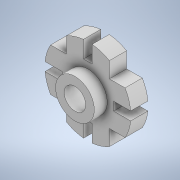
# Autodesk Inventor part: Assignment 3.5 - Indexing Guide
Saved by Autodesk Inventor 2022 (Build 260153000, 153)
## iProperties
Created: 2021-05-24
Part Number: Assignment 3.5 - Indexing Guide
Material: Generic
Document SubType Name: Modeling
Designer: Aaron
Density: 1 g/cm^3
Appearance: Default
Author: Aaron
Autodesk Inventor part; units mm, degrees
ref_plane "YZ Plane" through (0, 0, 0) normal (1, 0, 0) x (0, 1, 0)
ref_plane "XZ Plane" through (0, 0, 0) normal (0, 1, 0) x (-1, 0, 0)
ref_plane "XY Plane" through (0, 0, 0) normal (0, 0, 1) x (1, 0, 0)
sketch "Sketch1" plane through (0, 0, 0) normal (0, 0, 1) x (1, 0, 0)
  circle A0 centre (0, 0) radius 15.875
  line L0 (-38.1, 0) -> (-38.1, -6.35)
  line L1 (-38.1, 0) -> (-38.1, 6.35)
  line L2 (38.1, 0) -> (38.1, 6.35)
  line L3 (38.1, 0) -> (38.1, -6.35)
  line L4 (-38.1, 6.35) -> (-63.1817, 6.35)
  line L5 (-38.1, -6.35) -> (-63.1817, -6.35)
  line L6 (38.1, 6.35) -> (63.1817, 6.35)
  line L7 (38.1, -6.35) -> (63.1817, -6.35)
  line L8 (0, 38.1) -> (6.35, 38.1)
  line L9 (6.35, 38.1) -> (6.35, 63.1817)
  line L10 (0, 38.1) -> (-6.35, 38.1)
  line L11 (-6.35, 38.1) -> (-6.35, 63.1817)
  line L12 (0, 0) -> (0, -38.1)
  line L13 (0, -38.1) -> (6.35, -38.1)
  line L14 (0, -38.1) -> (-6.35, -38.1)
  line L15 (-6.35, -38.1) -> (-6.35, -63.1817)
  line L16 (6.35, -38.1) -> (6.35, -63.1817)
  line L17 (-31.75, 38.1) -> (-31.75, 54.9926)
  line L18 (31.75, 38.1) -> (31.75, 54.9926)
  line L19 (38.1, 31.75) -> (54.9926, 31.75)
  line L20 (38.1, -31.75) -> (54.9926, -31.75)
  line L21 (31.75, -38.1) -> (31.75, -54.9926)
  line L22 (-31.75, -38.1) -> (-31.75, -54.9926)
  line L23 (-38.1, 31.75) -> (-54.9926, 31.75)
  line L24 (-38.1, -31.75) -> (-54.9926, -31.75)
  line L25 (-38.1, -31.75) -> (-31.75, -31.75)
  line L26 (-31.75, -31.75) -> (-31.75, -38.1)
  line L27 (31.75, -38.1) -> (31.75, -31.75)
  line L28 (31.75, -31.75) -> (38.1, -31.75)
  arc A1 (-6.35, 63.1817) -> (-31.75, 54.9926) centre (0, 0) ccw
  arc A2 (31.75, 54.9926) -> (6.35, 63.1817) centre (0, 0) ccw
  arc A3 (63.1817, 6.35) -> (54.9926, 31.75) centre (0, 0) ccw
  arc A4 (6.35, -63.1817) -> (31.75, -54.9926) centre (0, 0) ccw
  arc A5 (54.9926, -31.75) -> (63.1817, -6.35) centre (0, 0) ccw
  arc A6 (-31.75, -54.9926) -> (-6.35, -63.1817) centre (0, 0) ccw
  arc A7 (-54.9926, 31.75) -> (-63.1817, 6.35) centre (0, 0) ccw
  arc A8 (-63.1817, -6.35) -> (-54.9926, -31.75) centre (0, 0) ccw
  line L29 (31.75, 38.1) -> (31.75, 31.75)
  line L30 (31.75, 31.75) -> (38.1, 31.75)
  line L31 (-38.1, 31.75) -> (-31.75, 31.75)
  line L32 (-31.75, 31.75) -> (-31.75, 38.1)
  dimension "d6" = 31.75
  dimension "d7" = 38.1
  dimension "d8" = 38.1
  dimension "d9" = 6.35
  dimension "d10" = 6.35
  dimension "d11" = 6.35
  dimension "d12" = 6.35
  dimension "d14" = 6.35
  dimension "d15" = 6.35
  dimension "d16" = 38.1
  dimension "d17" = 6.35
  dimension "d18" = 25.4
  dimension "d19" = 25.4
  dimension "d20" = 25.4
  dimension "d22" = 25.4
  dimension "d23" = 25.4
  dimension "d24" = 25.4
  dimension "d25" = 25.4
  constraints: 66 end point, 16 point on circle, 9 centre point, 8 horizontal, 7 perpendicular, 7 vertical, 2 coincident, 1 point on line
  measures "d6" diameter of A0
  measures "d7" distance of L12.start L2.start
  measures "d8" distance of L12.start L0.start
  measures "d9" distance of L0.start L0.end
  measures "d10" distance of L0.start L1.end
  measures "d11" distance of L2.start L2.end
  measures "d12" distance of L2.start L3.end
  measures "d14" distance of L8.start L8.end
  measures "d15" distance of L8.start L10.end
  measures "d16" distance of L12.start L12.end
  measures "d17" distance of L12.end L14.end
  measures "d18" distance of L10.end L17.start
  measures "d19" distance of L8.end L18.start
  measures "d20" distance of L2.end L19.start
  measures "d22" distance of L13.end L21.start
  measures "d23" distance of L14.end L22.start
  measures "d24" distance of L1.end L23.start
  measures "d25" distance of L0.end L24.start
extrude "Extrusion1" add sketch "Sketch1" along normal blind 25.4
sketch "Sketch2" plane through (0, 0, 25.4) normal (0, 0, 1) x (1, 0, 0)
  circle A0 centre (0, 0) radius 15.875
  circle A1 centre (0, 0) radius 28.575
  dimension "d28" = 31.75
  dimension "d29" = 57.15
  constraints: 2 centre point, 2 coincident
  measures "d28" diameter of A0
  measures "d29" diameter of A1
extrude "Extrusion2" add sketch "Sketch2" along normal blind 19.05
body "Solid1"
